Autodesk Fusion 360 part; units mm, degrees
(part 3 of 3)
  line L1634 (-109.9333, 31.86) -> (-100.9333, 31.86)
  line L1635 (-109.3333, 37.76) -> (-109.3333, 32.46)
  line L1636 (-101.5333, 37.76) -> (-109.3333, 37.76)
  line L1637 (-101.5333, 32.46) -> (-101.5333, 37.76)
  line L1638 (-119.1867, 32.46) -> (-111.3867, 32.46)
  line L1639 (-110.7867, 38.36) -> (-119.7867, 38.36)
  line L1640 (-119.7867, 38.36) -> (-119.7867, 31.86)
  line L1641 (-110.7867, 31.86) -> (-110.7867, 38.36)
  line L1642 (-119.7867, 31.86) -> (-110.7867, 31.86)
  line L1643 (-119.1867, 37.76) -> (-119.1867, 32.46)
  line L1644 (-111.3867, 37.76) -> (-119.1867, 37.76)
  line L1645 (-111.3867, 32.46) -> (-111.3867, 37.76)
  line L1646 (-129.04, 32.46) -> (-121.24, 32.46)
  line L1647 (-120.64, 38.36) -> (-129.64, 38.36)
  line L1648 (-129.64, 38.36) -> (-129.64, 31.86)
  line L1649 (-120.64, 31.86) -> (-120.64, 38.36)
  line L1650 (-129.64, 31.86) -> (-120.64, 31.86)
  line L1651 (-129.04, 37.76) -> (-129.04, 32.46)
  line L1652 (-121.24, 37.76) -> (-129.04, 37.76)
  line L1653 (-121.24, 32.46) -> (-121.24, 37.76)
  line L1654 (-138.8933, 32.46) -> (-131.0933, 32.46)
  line L1655 (-130.4933, 38.36) -> (-139.4933, 38.36)
  line L1656 (-139.4933, 38.36) -> (-139.4933, 31.86)
  line L1657 (-130.4933, 31.86) -> (-130.4933, 38.36)
  line L1658 (-139.4933, 31.86) -> (-130.4933, 31.86)
  line L1659 (-138.8933, 37.76) -> (-138.8933, 32.46)
  line L1660 (-131.0933, 37.76) -> (-138.8933, 37.76)
  line L1661 (-131.0933, 32.46) -> (-131.0933, 37.76)
  line L1662 (-148.7467, 32.46) -> (-140.9467, 32.46)
  line L1663 (-140.3467, 38.36) -> (-149.3467, 38.36)
  line L1664 (-149.3467, 38.36) -> (-149.3467, 31.86)
  line L1665 (-140.3467, 31.86) -> (-140.3467, 38.36)
  line L1666 (-149.3467, 31.86) -> (-140.3467, 31.86)
  line L1667 (-148.7467, 37.76) -> (-148.7467, 32.46)
  line L1668 (-140.9467, 37.76) -> (-148.7467, 37.76)
  line L1669 (-140.9467, 32.46) -> (-140.9467, 37.76)
  line L1670 (-158.6, 32.46) -> (-150.8, 32.46)
  line L1671 (-150.2, 38.36) -> (-159.2, 38.36)
  line L1672 (-159.2, 38.36) -> (-159.2, 31.86)
  line L1673 (-150.2, 31.86) -> (-150.2, 38.36)
  line L1674 (-159.2, 31.86) -> (-150.2, 31.86)
  line L1675 (-158.6, 37.76) -> (-158.6, 32.46)
  line L1676 (-150.8, 37.76) -> (-158.6, 37.76)
  line L1677 (-150.8, 32.46) -> (-150.8, 37.76)
  line L1678 (-10.8, 22.44) -> (-3, 22.44)
  line L1679 (-2.4, 28.34) -> (-11.4, 28.34)
  line L1680 (-11.4, 28.34) -> (-11.4, 21.84)
  line L1681 (-2.4, 21.84) -> (-2.4, 28.34)
  line L1682 (-11.4, 21.84) -> (-2.4, 21.84)
  line L1683 (-10.8, 27.74) -> (-10.8, 22.44)
  line L1684 (-3, 27.74) -> (-10.8, 27.74)
  line L1685 (-3, 22.44) -> (-3, 27.74)
  line L1686 (-20.6533, 22.44) -> (-12.8533, 22.44)
  line L1687 (-12.2533, 28.34) -> (-21.2533, 28.34)
  line L1688 (-21.2533, 28.34) -> (-21.2533, 21.84)
  line L1689 (-12.2533, 21.84) -> (-12.2533, 28.34)
  line L1690 (-21.2533, 21.84) -> (-12.2533, 21.84)
  line L1691 (-20.6533, 27.74) -> (-20.6533, 22.44)
  line L1692 (-12.8533, 27.74) -> (-20.6533, 27.74)
  line L1693 (-12.8533, 22.44) -> (-12.8533, 27.74)
  line L1694 (-30.5067, 22.44) -> (-22.7067, 22.44)
  line L1695 (-22.1067, 28.34) -> (-31.1067, 28.34)
  line L1696 (-31.1067, 28.34) -> (-31.1067, 21.84)
  line L1697 (-22.1067, 21.84) -> (-22.1067, 28.34)
  line L1698 (-31.1067, 21.84) -> (-22.1067, 21.84)
  line L1699 (-30.5067, 27.74) -> (-30.5067, 22.44)
  line L1700 (-22.7067, 27.74) -> (-30.5067, 27.74)
  line L1701 (-22.7067, 22.44) -> (-22.7067, 27.74)
  line L1702 (-40.36, 22.44) -> (-32.56, 22.44)
  line L1703 (-31.96, 28.34) -> (-40.96, 28.34)
  line L1704 (-40.96, 28.34) -> (-40.96, 21.84)
  line L1705 (-31.96, 21.84) -> (-31.96, 28.34)
  line L1706 (-40.96, 21.84) -> (-31.96, 21.84)
  line L1707 (-40.36, 27.74) -> (-40.36, 22.44)
  line L1708 (-32.56, 27.74) -> (-40.36, 27.74)
  line L1709 (-32.56, 22.44) -> (-32.56, 27.74)
  line L1710 (-50.2133, 22.44) -> (-42.4133, 22.44)
  line L1711 (-41.8133, 28.34) -> (-50.8133, 28.34)
  line L1712 (-50.8133, 28.34) -> (-50.8133, 21.84)
  line L1713 (-41.8133, 21.84) -> (-41.8133, 28.34)
  line L1714 (-50.8133, 21.84) -> (-41.8133, 21.84)
  line L1715 (-50.2133, 27.74) -> (-50.2133, 22.44)
  line L1716 (-42.4133, 27.74) -> (-50.2133, 27.74)
  line L1717 (-42.4133, 22.44) -> (-42.4133, 27.74)
  line L1718 (-60.0667, 22.44) -> (-52.2667, 22.44)
  line L1719 (-51.6667, 28.34) -> (-60.6667, 28.34)
  line L1720 (-60.6667, 28.34) -> (-60.6667, 21.84)
  line L1721 (-51.6667, 21.84) -> (-51.6667, 28.34)
  line L1722 (-60.6667, 21.84) -> (-51.6667, 21.84)
  line L1723 (-60.0667, 27.74) -> (-60.0667, 22.44)
  line L1724 (-52.2667, 27.74) -> (-60.0667, 27.74)
  line L1725 (-52.2667, 22.44) -> (-52.2667, 27.74)
  line L1726 (-69.92, 22.44) -> (-62.12, 22.44)
  line L1727 (-61.52, 28.34) -> (-70.52, 28.34)
  line L1728 (-70.52, 28.34) -> (-70.52, 21.84)
  line L1729 (-61.52, 21.84) -> (-61.52, 28.34)
  line L1730 (-70.52, 21.84) -> (-61.52, 21.84)
  line L1731 (-69.92, 27.74) -> (-69.92, 22.44)
  line L1732 (-62.12, 27.74) -> (-69.92, 27.74)
  line L1733 (-62.12, 22.44) -> (-62.12, 27.74)
  line L1734 (-79.7733, 22.44) -> (-71.9733, 22.44)
  line L1735 (-71.3733, 28.34) -> (-80.3733, 28.34)
  line L1736 (-80.3733, 28.34) -> (-80.3733, 21.84)
  line L1737 (-71.3733, 21.84) -> (-71.3733, 28.34)
  line L1738 (-80.3733, 21.84) -> (-71.3733, 21.84)
  line L1739 (-79.7733, 27.74) -> (-79.7733, 22.44)
  line L1740 (-71.9733, 27.74) -> (-79.7733, 27.74)
  line L1741 (-71.9733, 22.44) -> (-71.9733, 27.74)
  line L1742 (-89.6267, 22.44) -> (-81.8267, 22.44)
  line L1743 (-81.2267, 28.34) -> (-90.2267, 28.34)
  line L1744 (-90.2267, 28.34) -> (-90.2267, 21.84)
  line L1745 (-81.2267, 21.84) -> (-81.2267, 28.34)
  line L1746 (-90.2267, 21.84) -> (-81.2267, 21.84)
  line L1747 (-89.6267, 27.74) -> (-89.6267, 22.44)
  line L1748 (-81.8267, 27.74) -> (-89.6267, 27.74)
  line L1749 (-81.8267, 22.44) -> (-81.8267, 27.74)
  line L1750 (-99.48, 22.44) -> (-91.68, 22.44)
  line L1751 (-91.08, 28.34) -> (-100.08, 28.34)
  line L1752 (-100.08, 28.34) -> (-100.08, 21.84)
  line L1753 (-91.08, 21.84) -> (-91.08, 28.34)
  line L1754 (-100.08, 21.84) -> (-91.08, 21.84)
  line L1755 (-99.48, 27.74) -> (-99.48, 22.44)
  line L1756 (-91.68, 27.74) -> (-99.48, 27.74)
  line L1757 (-91.68, 22.44) -> (-91.68, 27.74)
  line L1758 (-109.3333, 22.44) -> (-101.5333, 22.44)
  line L1759 (-100.9333, 28.34) -> (-109.9333, 28.34)
  line L1760 (-109.9333, 28.34) -> (-109.9333, 21.84)
  line L1761 (-100.9333, 21.84) -> (-100.9333, 28.34)
  line L1762 (-109.9333, 21.84) -> (-100.9333, 21.84)
  line L1763 (-109.3333, 27.74) -> (-109.3333, 22.44)
  line L1764 (-101.5333, 27.74) -> (-109.3333, 27.74)
  line L1765 (-101.5333, 22.44) -> (-101.5333, 27.74)
  line L1766 (-119.1867, 22.44) -> (-111.3867, 22.44)
  line L1767 (-110.7867, 28.34) -> (-119.7867, 28.34)
  line L1768 (-119.7867, 28.34) -> (-119.7867, 21.84)
  line L1769 (-110.7867, 21.84) -> (-110.7867, 28.34)
  line L1770 (-119.7867, 21.84) -> (-110.7867, 21.84)
  line L1771 (-119.1867, 27.74) -> (-119.1867, 22.44)
  line L1772 (-111.3867, 27.74) -> (-119.1867, 27.74)
  line L1773 (-111.3867, 22.44) -> (-111.3867, 27.74)
  line L1774 (-129.04, 22.44) -> (-121.24, 22.44)
  line L1775 (-120.64, 28.34) -> (-129.64, 28.34)
  line L1776 (-129.64, 28.34) -> (-129.64, 21.84)
  line L1777 (-120.64, 21.84) -> (-120.64, 28.34)
  line L1778 (-129.64, 21.84) -> (-120.64, 21.84)
  line L1779 (-129.04, 27.74) -> (-129.04, 22.44)
  line L1780 (-121.24, 27.74) -> (-129.04, 27.74)
  line L1781 (-121.24, 22.44) -> (-121.24, 27.74)
  line L1782 (-138.8933, 22.44) -> (-131.0933, 22.44)
  line L1783 (-130.4933, 28.34) -> (-139.4933, 28.34)
  line L1784 (-139.4933, 28.34) -> (-139.4933, 21.84)
  line L1785 (-130.4933, 21.84) -> (-130.4933, 28.34)
  line L1786 (-139.4933, 21.84) -> (-130.4933, 21.84)
  line L1787 (-138.8933, 27.74) -> (-138.8933, 22.44)
  line L1788 (-131.0933, 27.74) -> (-138.8933, 27.74)
  line L1789 (-131.0933, 22.44) -> (-131.0933, 27.74)
  line L1790 (-148.7467, 22.44) -> (-140.9467, 22.44)
  line L1791 (-140.3467, 28.34) -> (-149.3467, 28.34)
  line L1792 (-149.3467, 28.34) -> (-149.3467, 21.84)
  line L1793 (-140.3467, 21.84) -> (-140.3467, 28.34)
  line L1794 (-149.3467, 21.84) -> (-140.3467, 21.84)
  line L1795 (-148.7467, 27.74) -> (-148.7467, 22.44)
  line L1796 (-140.9467, 27.74) -> (-148.7467, 27.74)
  line L1797 (-140.9467, 22.44) -> (-140.9467, 27.74)
  line L1798 (-158.6, 22.44) -> (-150.8, 22.44)
  line L1799 (-150.2, 28.34) -> (-159.2, 28.34)
  line L1800 (-159.2, 28.34) -> (-159.2, 21.84)
  line L1801 (-150.2, 21.84) -> (-150.2, 28.34)
  line L1802 (-159.2, 21.84) -> (-150.2, 21.84)
  line L1803 (-158.6, 27.74) -> (-158.6, 22.44)
  line L1804 (-150.8, 27.74) -> (-158.6, 27.74)
  line L1805 (-150.8, 22.44) -> (-150.8, 27.74)
  line L1806 (-10.8, 12.42) -> (-3, 12.42)
  line L1807 (-2.4, 18.32) -> (-11.4, 18.32)
  line L1808 (-11.4, 18.32) -> (-11.4, 11.82)
  line L1809 (-2.4, 11.82) -> (-2.4, 18.32)
  line L1810 (-11.4, 11.82) -> (-2.4, 11.82)
  line L1811 (-10.8, 17.72) -> (-10.8, 12.42)
  line L1812 (-3, 17.72) -> (-10.8, 17.72)
  line L1813 (-3, 12.42) -> (-3, 17.72)
  line L1814 (-20.6533, 12.42) -> (-12.8533, 12.42)
  line L1815 (-12.2533, 18.32) -> (-21.2533, 18.32)
  line L1816 (-21.2533, 18.32) -> (-21.2533, 11.82)
  line L1817 (-12.2533, 11.82) -> (-12.2533, 18.32)
  line L1818 (-21.2533, 11.82) -> (-12.2533, 11.82)
  line L1819 (-20.6533, 17.72) -> (-20.6533, 12.42)
  line L1820 (-12.8533, 17.72) -> (-20.6533, 17.72)
  line L1821 (-12.8533, 12.42) -> (-12.8533, 17.72)
  line L1822 (-30.5067, 12.42) -> (-22.7067, 12.42)
  line L1823 (-22.1067, 18.32) -> (-31.1067, 18.32)
  line L1824 (-31.1067, 18.32) -> (-31.1067, 11.82)
  line L1825 (-22.1067, 11.82) -> (-22.1067, 18.32)
  line L1826 (-31.1067, 11.82) -> (-22.1067, 11.82)
  line L1827 (-30.5067, 17.72) -> (-30.5067, 12.42)
  line L1828 (-22.7067, 17.72) -> (-30.5067, 17.72)
  line L1829 (-22.7067, 12.42) -> (-22.7067, 17.72)
  line L1830 (-40.36, 12.42) -> (-32.56, 12.42)
  line L1831 (-31.96, 18.32) -> (-40.96, 18.32)
  line L1832 (-40.96, 18.32) -> (-40.96, 11.82)
  line L1833 (-31.96, 11.82) -> (-31.96, 18.32)
  line L1834 (-40.96, 11.82) -> (-31.96, 11.82)
  line L1835 (-40.36, 17.72) -> (-40.36, 12.42)
  line L1836 (-32.56, 17.72) -> (-40.36, 17.72)
  line L1837 (-32.56, 12.42) -> (-32.56, 17.72)
  line L1838 (-50.2133, 12.42) -> (-42.4133, 12.42)
  line L1839 (-41.8133, 18.32) -> (-50.8133, 18.32)
  line L1840 (-50.8133, 18.32) -> (-50.8133, 11.82)
  line L1841 (-41.8133, 11.82) -> (-41.8133, 18.32)
  line L1842 (-50.8133, 11.82) -> (-41.8133, 11.82)
  line L1843 (-50.2133, 17.72) -> (-50.2133, 12.42)
  line L1844 (-42.4133, 17.72) -> (-50.2133, 17.72)
  line L1845 (-42.4133, 12.42) -> (-42.4133, 17.72)
  line L1846 (-60.0667, 12.42) -> (-52.2667, 12.42)
  line L1847 (-51.6667, 18.32) -> (-60.6667, 18.32)
  line L1848 (-60.6667, 18.32) -> (-60.6667, 11.82)
  line L1849 (-51.6667, 11.82) -> (-51.6667, 18.32)
  line L1850 (-60.6667, 11.82) -> (-51.6667, 11.82)
  line L1851 (-60.0667, 17.72) -> (-60.0667, 12.42)
  line L1852 (-52.2667, 17.72) -> (-60.0667, 17.72)
  line L1853 (-52.2667, 12.42) -> (-52.2667, 17.72)
  line L1854 (-69.92, 12.42) -> (-62.12, 12.42)
  line L1855 (-61.52, 18.32) -> (-70.52, 18.32)
  line L1856 (-70.52, 18.32) -> (-70.52, 11.82)
  line L1857 (-61.52, 11.82) -> (-61.52, 18.32)
  line L1858 (-70.52, 11.82) -> (-61.52, 11.82)
  line L1859 (-69.92, 17.72) -> (-69.92, 12.42)
  line L1860 (-62.12, 17.72) -> (-69.92, 17.72)
  line L1861 (-62.12, 12.42) -> (-62.12, 17.72)
  line L1862 (-79.7733, 12.42) -> (-71.9733, 12.42)
  line L1863 (-71.3733, 18.32) -> (-80.3733, 18.32)
  line L1864 (-80.3733, 18.32) -> (-80.3733, 11.82)
  line L1865 (-71.3733, 11.82) -> (-71.3733, 18.32)
  line L1866 (-80.3733, 11.82) -> (-71.3733, 11.82)
  line L1867 (-79.7733, 17.72) -> (-79.7733, 12.42)
  line L1868 (-71.9733, 17.72) -> (-79.7733, 17.72)
  line L1869 (-71.9733, 12.42) -> (-71.9733, 17.72)
  line L1870 (-89.6267, 12.42) -> (-81.8267, 12.42)
  line L1871 (-81.2267, 18.32) -> (-90.2267, 18.32)
  line L1872 (-90.2267, 18.32) -> (-90.2267, 11.82)
  line L1873 (-81.2267, 11.82) -> (-81.2267, 18.32)
  line L1874 (-90.2267, 11.82) -> (-81.2267, 11.82)
  line L1875 (-89.6267, 17.72) -> (-89.6267, 12.42)
  line L1876 (-81.8267, 17.72) -> (-89.6267, 17.72)
  line L1877 (-81.8267, 12.42) -> (-81.8267, 17.72)
  line L1878 (-99.48, 12.42) -> (-91.68, 12.42)
  line L1879 (-91.08, 18.32) -> (-100.08, 18.32)
  line L1880 (-100.08, 18.32) -> (-100.08, 11.82)
  line L1881 (-91.08, 11.82) -> (-91.08, 18.32)
  line L1882 (-100.08, 11.82) -> (-91.08, 11.82)
  line L1883 (-99.48, 17.72) -> (-99.48, 12.42)
  line L1884 (-91.68, 17.72) -> (-99.48, 17.72)
  line L1885 (-91.68, 12.42) -> (-91.68, 17.72)
  line L1886 (-109.3333, 12.42) -> (-101.5333, 12.42)
  line L1887 (-100.9333, 18.32) -> (-109.9333, 18.32)
  line L1888 (-109.9333, 18.32) -> (-109.9333, 11.82)
  line L1889 (-100.9333, 11.82) -> (-100.9333, 18.32)
  line L1890 (-109.9333, 11.82) -> (-100.9333, 11.82)
  line L1891 (-109.3333, 17.72) -> (-109.3333, 12.42)
  line L1892 (-101.5333, 17.72) -> (-109.3333, 17.72)
  line L1893 (-101.5333, 12.42) -> (-101.5333, 17.72)
  line L1894 (-119.1867, 12.42) -> (-111.3867, 12.42)
  line L1895 (-110.7867, 18.32) -> (-119.7867, 18.32)
  line L1896 (-119.7867, 18.32) -> (-119.7867, 11.82)
  line L1897 (-110.7867, 11.82) -> (-110.7867, 18.32)
  line L1898 (-119.7867, 11.82) -> (-110.7867, 11.82)
  line L1899 (-119.1867, 17.72) -> (-119.1867, 12.42)
  line L1900 (-111.3867, 17.72) -> (-119.1867, 17.72)
  line L1901 (-111.3867, 12.42) -> (-111.3867, 17.72)
  line L1902 (-129.04, 12.42) -> (-121.24, 12.42)
  line L1903 (-120.64, 18.32) -> (-129.64, 18.32)
  line L1904 (-129.64, 18.32) -> (-129.64, 11.82)
  line L1905 (-120.64, 11.82) -> (-120.64, 18.32)
  line L1906 (-129.64, 11.82) -> (-120.64, 11.82)
  line L1907 (-129.04, 17.72) -> (-129.04, 12.42)
  line L1908 (-121.24, 17.72) -> (-129.04, 17.72)
  line L1909 (-121.24, 12.42) -> (-121.24, 17.72)
  line L1910 (-138.8933, 12.42) -> (-131.0933, 12.42)
  line L1911 (-130.4933, 18.32) -> (-139.4933, 18.32)
  line L1912 (-139.4933, 18.32) -> (-139.4933, 11.82)
  line L1913 (-130.4933, 11.82) -> (-130.4933, 18.32)
  line L1914 (-139.4933, 11.82) -> (-130.4933, 11.82)
  line L1915 (-138.8933, 17.72) -> (-138.8933, 12.42)
  line L1916 (-131.0933, 17.72) -> (-138.8933, 17.72)
  line L1917 (-131.0933, 12.42) -> (-131.0933, 17.72)
  line L1918 (-148.7467, 12.42) -> (-140.9467, 12.42)
  line L1919 (-140.3467, 18.32) -> (-149.3467, 18.32)
  line L1920 (-149.3467, 18.32) -> (-149.3467, 11.82)
  line L1921 (-140.3467, 11.82) -> (-140.3467, 18.32)
  line L1922 (-149.3467, 11.82) -> (-140.3467, 11.82)
  line L1923 (-148.7467, 17.72) -> (-148.7467, 12.42)
  line L1924 (-140.9467, 17.72) -> (-148.7467, 17.72)
  line L1925 (-140.9467, 12.42) -> (-140.9467, 17.72)
  line L1926 (-158.6, 12.42) -> (-150.8, 12.42)
  line L1927 (-150.2, 18.32) -> (-159.2, 18.32)
  line L1928 (-159.2, 18.32) -> (-159.2, 11.82)
  line L1929 (-150.2, 11.82) -> (-150.2, 18.32)
  line L1930 (-159.2, 11.82) -> (-150.2, 11.82)
  line L1931 (-158.6, 17.72) -> (-158.6, 12.42)
  line L1932 (-150.8, 17.72) -> (-158.6, 17.72)
  line L1933 (-150.8, 12.42) -> (-150.8, 17.72)
  line L1934 (-10.8, 2.4) -> (-3, 2.4)
  line L1935 (-2.4, 8.3) -> (-11.4, 8.3)
  line L1936 (-11.4, 8.3) -> (-11.4, 1.8)
  line L1937 (-2.4, 1.8) -> (-2.4, 8.3)
  line L1938 (-11.4, 1.8) -> (-2.4, 1.8)
  line L1939 (-10.8, 7.7) -> (-10.8, 2.4)
  line L1940 (-3, 7.7) -> (-10.8, 7.7)
  line L1941 (-3, 2.4) -> (-3, 7.7)
  line L1942 (-20.6533, 2.4) -> (-12.8533, 2.4)
  line L1943 (-12.2533, 8.3) -> (-21.2533, 8.3)
  line L1944 (-21.2533, 8.3) -> (-21.2533, 1.8)
  line L1945 (-12.2533, 1.8) -> (-12.2533, 8.3)
  line L1946 (-21.2533, 1.8) -> (-12.2533, 1.8)
  line L1947 (-20.6533, 7.7) -> (-20.6533, 2.4)
  line L1948 (-12.8533, 7.7) -> (-20.6533, 7.7)
  line L1949 (-12.8533, 2.4) -> (-12.8533, 7.7)
  line L1950 (-30.5067, 2.4) -> (-22.7067, 2.4)
  line L1951 (-22.1067, 8.3) -> (-31.1067, 8.3)
  line L1952 (-31.1067, 8.3) -> (-31.1067, 1.8)
  line L1953 (-22.1067, 1.8) -> (-22.1067, 8.3)
  line L1954 (-31.1067, 1.8) -> (-22.1067, 1.8)
  line L1955 (-30.5067, 7.7) -> (-30.5067, 2.4)
  line L1956 (-22.7067, 7.7) -> (-30.5067, 7.7)
  line L1957 (-22.7067, 2.4) -> (-22.7067, 7.7)
  line L1958 (-40.36, 2.4) -> (-32.56, 2.4)
  line L1959 (-31.96, 8.3) -> (-40.96, 8.3)
  line L1960 (-40.96, 8.3) -> (-40.96, 1.8)
  line L1961 (-31.96, 1.8) -> (-31.96, 8.3)
  line L1962 (-40.96, 1.8) -> (-31.96, 1.8)
  line L1963 (-40.36, 7.7) -> (-40.36, 2.4)
  line L1964 (-32.56, 7.7) -> (-40.36, 7.7)
  line L1965 (-32.56, 2.4) -> (-32.56, 7.7)
  line L1966 (-50.2133, 2.4) -> (-42.4133, 2.4)
  line L1967 (-41.8133, 8.3) -> (-50.8133, 8.3)
  line L1968 (-50.8133, 8.3) -> (-50.8133, 1.8)
  line L1969 (-41.8133, 1.8) -> (-41.8133, 8.3)
  line L1970 (-50.8133, 1.8) -> (-41.8133, 1.8)
  line L1971 (-50.2133, 7.7) -> (-50.2133, 2.4)
  line L1972 (-42.4133, 7.7) -> (-50.2133, 7.7)
  line L1973 (-42.4133, 2.4) -> (-42.4133, 7.7)
  line L1974 (-60.0667, 2.4) -> (-52.2667, 2.4)
  line L1975 (-51.6667, 8.3) -> (-60.6667, 8.3)
  line L1976 (-60.6667, 8.3) -> (-60.6667, 1.8)
  line L1977 (-51.6667, 1.8) -> (-51.6667, 8.3)
  line L1978 (-60.6667, 1.8) -> (-51.6667, 1.8)
  line L1979 (-60.0667, 7.7) -> (-60.0667, 2.4)
  line L1980 (-52.2667, 7.7) -> (-60.0667, 7.7)
  line L1981 (-52.2667, 2.4) -> (-52.2667, 7.7)
  line L1982 (-69.92, 2.4) -> (-62.12, 2.4)
  line L1983 (-61.52, 8.3) -> (-70.52, 8.3)
  line L1984 (-70.52, 8.3) -> (-70.52, 1.8)
  line L1985 (-61.52, 1.8) -> (-61.52, 8.3)
  line L1986 (-70.52, 1.8) -> (-61.52, 1.8)
  line L1987 (-69.92, 7.7) -> (-69.92, 2.4)
  line L1988 (-62.12, 7.7) -> (-69.92, 7.7)
  line L1989 (-62.12, 2.4) -> (-62.12, 7.7)
  line L1990 (-79.7733, 2.4) -> (-71.9733, 2.4)
  line L1991 (-71.3733, 8.3) -> (-80.3733, 8.3)
  line L1992 (-80.3733, 8.3) -> (-80.3733, 1.8)
  line L1993 (-71.3733, 1.8) -> (-71.3733, 8.3)
  line L1994 (-80.3733, 1.8) -> (-71.3733, 1.8)
  line L1995 (-79.7733, 7.7) -> (-79.7733, 2.4)
  line L1996 (-71.9733, 7.7) -> (-79.7733, 7.7)
  line L1997 (-71.9733, 2.4) -> (-71.9733, 7.7)
  line L1998 (-89.6267, 2.4) -> (-81.8267, 2.4)
  line L1999 (-81.2267, 8.3) -> (-90.2267, 8.3)
  line L2000 (-90.2267, 8.3) -> (-90.2267, 1.8)
  line L2001 (-81.2267, 1.8) -> (-81.2267, 8.3)
  line L2002 (-90.2267, 1.8) -> (-81.2267, 1.8)
  line L2003 (-89.6267, 7.7) -> (-89.6267, 2.4)
  line L2004 (-81.8267, 7.7) -> (-89.6267, 7.7)
  line L2005 (-81.8267, 2.4) -> (-81.8267, 7.7)
  line L2006 (-99.48, 2.4) -> (-91.68, 2.4)
  line L2007 (-91.08, 8.3) -> (-100.08, 8.3)
  line L2008 (-100.08, 8.3) -> (-100.08, 1.8)
  line L2009 (-91.08, 1.8) -> (-91.08, 8.3)
  line L2010 (-100.08, 1.8) -> (-91.08, 1.8)
  line L2011 (-99.48, 7.7) -> (-99.48, 2.4)
  line L2012 (-91.68, 7.7) -> (-99.48, 7.7)
  line L2013 (-91.68, 2.4) -> (-91.68, 7.7)
  line L2014 (-109.3333, 2.4) -> (-101.5333, 2.4)
  line L2015 (-100.9333, 8.3) -> (-109.9333, 8.3)
  line L2016 (-109.9333, 8.3) -> (-109.9333, 1.8)
  line L2017 (-100.9333, 1.8) -> (-100.9333, 8.3)
  line L2018 (-109.9333, 1.8) -> (-100.9333, 1.8)
  line L2019 (-109.3333, 7.7) -> (-109.3333, 2.4)
  line L2020 (-101.5333, 7.7) -> (-109.3333, 7.7)
  line L2021 (-101.5333, 2.4) -> (-101.5333, 7.7)
  line L2022 (-119.1867, 2.4) -> (-111.3867, 2.4)
  line L2023 (-110.7867, 8.3) -> (-119.7867, 8.3)
  line L2024 (-119.7867, 8.3) -> (-119.7867, 1.8)
  line L2025 (-110.7867, 1.8) -> (-110.7867, 8.3)
  line L2026 (-119.7867, 1.8) -> (-110.7867, 1.8)
  line L2027 (-119.1867, 7.7) -> (-119.1867, 2.4)
  line L2028 (-111.3867, 7.7) -> (-119.1867, 7.7)
  line L2029 (-111.3867, 2.4) -> (-111.3867, 7.7)
  line L2030 (-129.04, 2.4) -> (-121.24, 2.4)
  line L2031 (-120.64, 8.3) -> (-129.64, 8.3)
  line L2032 (-129.64, 8.3) -> (-129.64, 1.8)
  line L2033 (-120.64, 1.8) -> (-120.64, 8.3)
  line L2034 (-129.64, 1.8) -> (-120.64, 1.8)
  line L2035 (-129.04, 7.7) -> (-129.04, 2.4)
  line L2036 (-121.24, 7.7) -> (-129.04, 7.7)
  line L2037 (-121.24, 2.4) -> (-121.24, 7.7)
  line L2038 (-138.8933, 2.4) -> (-131.0933, 2.4)
  line L2039 (-130.4933, 8.3) -> (-139.4933, 8.3)
  line L2040 (-139.4933, 8.3) -> (-139.4933, 1.8)
  line L2041 (-130.4933, 1.8) -> (-130.4933, 8.3)
  line L2042 (-139.4933, 1.8) -> (-130.4933, 1.8)
  line L2043 (-138.8933, 7.7) -> (-138.8933, 2.4)
  line L2044 (-131.0933, 7.7) -> (-138.8933, 7.7)
  line L2045 (-131.0933, 2.4) -> (-131.0933, 7.7)
  line L2046 (-148.7467, 2.4) -> (-140.9467, 2.4)
  line L2047 (-140.3467, 8.3) -> (-149.3467, 8.3)
  line L2048 (-149.3467, 8.3) -> (-149.3467, 1.8)
  line L2049 (-140.3467, 1.8) -> (-140.3467, 8.3)
  line L2050 (-149.3467, 1.8) -> (-140.3467, 1.8)
  line L2051 (-148.7467, 7.7) -> (-148.7467, 2.4)
  line L2052 (-140.9467, 7.7) -> (-148.7467, 7.7)
  line L2053 (-140.9467, 2.4) -> (-140.9467, 7.7)
  line L2054 (-158.6, 2.4) -> (-150.8, 2.4)
  line L2055 (-150.2, 8.3) -> (-159.2, 8.3)
  line L2056 (-159.2, 8.3) -> (-159.2, 1.8)
  line L2057 (-150.2, 1.8) -> (-150.2, 8.3)
  line L2058 (-159.2, 1.8) -> (-150.2, 1.8)
  line L2059 (-158.6, 7.7) -> (-158.6, 2.4)
  line L2060 (-150.8, 7.7) -> (-158.6, 7.7)
  line L2061 (-150.8, 2.4) -> (-150.8, 7.7)
  dimension "d58" = 156.2
  dimension "d59" = 2.4
  dimension "d60" = 2.4
  dimension "d61" = 156.2
  dimension "d62" = 9
  dimension "d63" = 6.5
  dimension "d64" = 0.6
  dimension "d65" = 0.6
  dimension "d66" = 7.8
  dimension "d67" = 5.3
  dimension "d70" = -147.8
  dimension "d71" = -150.3
  constraint horizontal L4
  constraint vertical L5
  constraint horizontal L6
  constraint vertical L7
  constraint coincident L1.end L2.start
  constraint perpendicular L5 L8
  constraint perpendicular L6 L9
  constraint horizontal L10
  constraint vertical L11
  constraint horizontal L12
  constraint vertical L13
  constraint horizontal L14
  constraint vertical L15
  constraint horizontal L16
  constraint vertical L17
  constraint horizontal L18
  constraint vertical L19
  constraint horizontal L20
  constraint vertical L21
  measures "d58" distance of L5.end L8.end
  measures "d59" distance of L5.end L6.end
  measures "d60" distance of L1.end L6.end
  measures "d61" distance of L5.end L9.end
  measures "d62" distance of L5.end L10.end
  measures "d63" distance of L10.end L11.end
  measures "d64" distance of L5.end L16.end
  measures "d65" distance of L5.end L14.end
  measures "d66" distance of L15.end L18.end
  measures "d67" distance of L18.end L19.end
extrude "Extrusion8" add sketch "Skizze4" along normal blind 1 contours L0 L1 L2 L3 bodies 3
chamfer "Fase1" distance 2 angle 45 6 edges at (11.9699, 86, -4) (11.9699, 76, -4) (11.9699, 46, -4) (11.9699, 36, -4) (11.9699, 116, -4) (11.9699, 126, -4) on bodies 2
chamfer "Fase1" distance 2 angle 45 3 edges at (45, 81, -4) (45, 41, -4) (45, 121, -4) on bodies 2
equation "d2 = d1"
equation "d3 = 4 * Nozzle"
equation "Nozzle = 0.6 mm"
equation "d5 = d3"
equation "d6 = d1 + 2 * d3"
equation "d7 = d6"
equation "d12 = d3"
equation "d13 = d12"
equation "d22 = d21"
equation "d23 = d21"
equation "d38 = -d6 + d35"
equation "d39 = d6 - d35"
equation "d42 = d3"
equation "d43 = d3"
equation "d44 = d1"
equation "d45 = d2"
equation "d58 = 155 mm + 2 * Nozzle"
equation "d59 = 3 mm - d64"
equation "d60 = d59"
equation "d61 = d58"
equation "d64 = Nozzle"
equation "d65 = d64"
equation "d66 = d62 - 2 * d65"
equation "d67 = d63 - 2 * d64"
equation "d70 = -156.2 mm + 9 mm - Nozzle"
equation "d71 = -156.2 mm + 6.5 mm - Nozzle"
equation "d74 = d21 + 3 * Nozzle"
equation "d75 = 3 * Nozzle"
named bodies: "Unterseite", "Diffuser"
